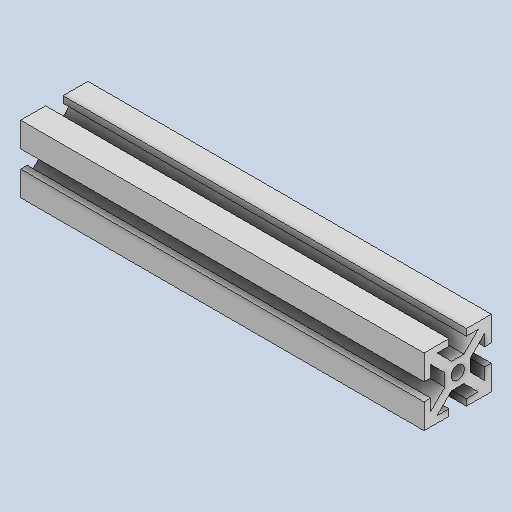
# Autodesk Inventor part: LatX24in1
Saved by Autodesk Inventor 2023 (Build 270158030, 158C)
## iProperties
Created: 2022-06-29
Part Number: LatX24in1
Material: Generic
Document SubType Name: Modeling
Designer: jeremyy
Density: 1 g/cm^3
Appearance: Default
Author: jeremyy
Autodesk Inventor part; units mm, degrees
ref_plane "YZ Plane" through (0, 0, 0) normal (1, 0, 0) x (0, 1, 0)
ref_plane "XZ Plane" through (0, 0, 0) normal (0, 1, 0) x (-1, 0, 0)
ref_plane "XY Plane" through (0, 0, 0) normal (0, 0, 1) x (1, 0, 0)
sketch "Sketch1" plane through (0, 0, 0) normal (1, 0, 0) x (0, 1, 0)
  line L0 (0, 0) -> (0, -9.398)
  line L1 (0, -9.398) -> (2.4765, -9.398)
  line L2 (9.398, -2.4765) -> (9.398, 0)
  line L3 (9.398, 0) -> (0, 0)
  line L4 (16.002, 0) -> (16.002, -2.4765)
  line L5 (22.9235, -9.398) -> (25.4, -9.398)
  line L6 (25.4, -9.398) -> (25.4, 0)
  line L7 (25.4, 0) -> (16.002, 0)
  line L8 (25.4, -16.002) -> (22.9235, -16.002)
  line L9 (16.002, -22.9235) -> (16.002, -25.4)
  line L10 (16.002, -25.4) -> (25.4, -25.4)
  line L11 (25.4, -25.4) -> (25.4, -16.002)
  line L12 (0, -16.002) -> (2.4765, -16.002)
  line L13 (9.398, -22.9235) -> (9.398, -25.4)
  line L14 (9.398, -25.4) -> (0, -25.4)
  line L15 (0, -25.4) -> (0, -16.002)
  line L16 (22.9235, -9.398) -> (22.9235, -4.953)
  line L17 (16.002, -2.4765) -> (20.447, -2.4765)
  line L18 (20.447, -2.4765) -> (15.0495, -7.874)
  line L19 (20.447, -2.4765) -> (28.0802, -2.4765) construction
  line L20 (22.9235, -4.953) -> (17.526, -10.3505)
  line L21 (22.9235, -16.002) -> (22.9235, -20.447)
  line L22 (22.9235, -20.447) -> (17.526, -15.0495)
  line L23 (16.002, -22.9235) -> (20.447, -22.9235)
  line L24 (20.447, -22.9235) -> (15.0495, -17.526)
  line L25 (2.4765, -16.002) -> (2.4765, -20.447)
  line L26 (2.4765, -20.447) -> (7.874, -15.0495)
  line L27 (9.398, -22.9235) -> (4.953, -22.9235)
  line L28 (4.953, -22.9235) -> (10.3505, -17.526)
  line L29 (9.398, -2.4765) -> (4.953, -2.4765)
  line L30 (4.953, -2.4765) -> (10.3505, -7.874)
  line L31 (2.4765, -9.398) -> (2.4765, -4.953)
  line L32 (2.4765, -4.953) -> (7.874, -10.3505)
  line L33 (10.3505, -7.874) -> (15.0495, -7.874)
  line L34 (17.526, -10.3505) -> (17.526, -15.0495)
  line L35 (10.3505, -17.526) -> (15.0495, -17.526)
  line L36 (7.874, -15.0495) -> (7.874, -10.3505)
  circle A0 centre (12.7, -12.7) radius 2.54
  dimension "d2" = 9.398
  dimension "d3" = 2.4765
  dimension "d7" = 2.4765
  dimension "d10" = 2.4765
  dimension "d11" = 25.4
  dimension "d13" = 2.4765
  dimension "d16" = 2.4765
  dimension "d17" = 9.398
  dimension "d18" = 25.4
  dimension "d23" = 2.4765
  dimension "d24" = 25.4
  dimension "d25" = 25.4
  dimension "d32" = 4.445
  dimension "d33" = 4.445
  dimension "d35" = 135
  dimension "d36" = 4.445
  dimension "d37" = 4.445
  dimension "d38" = 2.4765
  dimension "d40" = 4.445
  dimension "d41" = 4.445
  dimension "d42" = 4.445
  dimension "d43" = 4.445
  dimension "d44" = 5.08
  constraints: 74 end point, 12 perpendicular, 4 horizontal, 4 vertical, 3 parallel, 1 centre point, 1 equal length
  measures "d2" distance of L0.start L0.end
  measures "d3" distance of L0.end L1.end
  measures "d7" distance of L4.start L4.end
  measures "d10" distance of L5.start L5.end
  measures "d11" distance between parallel lines of L0 L6
  measures "d13" distance of L8.start L8.end
  measures "d16" distance of L9.start L9.end
  measures "d17" distance of L9.end L10.end
  measures "d18" distance between parallel lines of L10 L7
  measures "d23" distance of L13.start L13.end
  measures "d24" distance between parallel lines of L14 L3
  measures "d25" distance between parallel lines of L11 L15
  measures "d32" distance of L5.start L16.end
  measures "d33" distance of L4.end L17.end
  measures "d35" angle of L18 L19
  measures "d36" distance of L8.end L21.end
  measures "d37" distance of L9.start L23.end
  measures "d38" distance of L2.start L2.end
  measures "d40" distance of L12.end L25.end
  measures "d41" distance of L13.start L27.end
  measures "d42" distance of L2.start L29.end
  measures "d43" distance of L1.end L31.end
  measures "d44" diameter of A0
extrude "Extrusion1" add sketch "Sketch1" along normal blind 152.4
body "Solid1"
